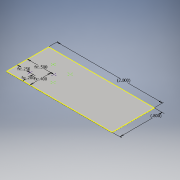
# Autodesk Inventor part: MAX Quarter-Scale Servo Frame Mounting Bracket
Saved by Autodesk Inventor 2016 (Build 200138000, 138)
## iProperties
Created: 2015-10-17
Part Number: MAX Quarter-Scale Servo Frame Mounting Bracket
Material: Generic
Document SubType Name: Modeling
Designer: Delta
Density: 1 g/cm^3
Appearance: Default
Author: Delta
Autodesk Inventor part; units mm, degrees
ref_plane "YZ Plane" through (0, 0, 0) normal (1, 0, 0) x (0, 1, 0)
ref_plane "XZ Plane" through (0, 0, 0) normal (0, 1, 0) x (-1, 0, 0)
ref_plane "XY Plane" through (0, 0, 0) normal (0, 0, 1) x (1, 0, 0)
sketch "Sketch1" plane through (0, 0, 0) normal (0, 1, 0) x (-1, 0, 0)
  line L0 (0, 0) -> (50.8, 0)
  line L1 (50.8, 0) -> (50.8, -20.32)
  line L2 (50.8, -20.32) -> (0, -20.32)
  line L3 (0, -20.32) -> (0, 0)
  dimension "d0" = 50.8
  dimension "d1" = 20.32
  constraints: 8 end point, 2 parallel, 1 horizontal, 1 perpendicular
  measures "d0" distance between parallel lines of L3 L1
  measures "d1" distance of L1.end L0.end
extrude "Extrusion1" add sketch "Sketch1" along normal blind 0.254
sketch "Sketch2" plane through (0, 0.254, 0) normal (0, 1, 0) x (1, 0, 0)
  line L0 (0, 0) -> (0, 20.32) projected
  line L1 (-50.8, 20.32) -> (-50.8, 0) projected
  line L2 (0, 20.32) -> (-50.8, 20.32) projected
  line L3 (-50.8, 0) -> (0, 0) projected
  point P0 (-38.1, 10.16)
  point P1 (-44.45, 5.08)
  point P2 (-42.3832, 14.1547)
  point P3 (-34.8233, 6.5948)
  point P4 (-34.1844, 14.1547)
  dimension "d4" = 50.8
  dimension "d7" = 20.32
  dimension "d9" = 12.7
  dimension "d10" = 10.16
  dimension "d11" = 5.08
  dimension "d12" = 6.35
  measures "d4" distance between parallel lines of L0 L1
  measures "d7" distance between parallel lines of L2 L3
  measures "d9" distance from line of point (-38.1, 10.16) L1
  measures "d10" distance from line of point (-38.1, 10.16) L3
  measures "d11" distance from line of point (-44.45, 5.08) L3
  measures "d12" distance from line of L1 point (-44.45, 5.08)
equation "\"d9\" = 0.25 * d4"
equation "\"d10\" = 0.5 * d7"
equation "\"d11\" = 0.5 * d10"
equation "\"d12\" = 0.5 * d9"
body "Solid1"
